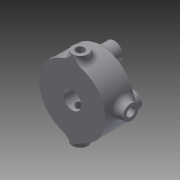
# Autodesk Inventor part: stick-holder-top
Saved by Autodesk Inventor 2014 (Build 180170000, 170)
## iProperties
Created: 2017-07-21
Part Number: stick-holder-top
Material: 一般
Document SubType Name: Modeling
Designer: hide
Density: 1 g/cm^3
Appearance: 既定
Author: hide
Autodesk Inventor part; units mm, degrees
ref_plane "YZ Plane" through (0, 0, 0) normal (1, 0, 0) x (0, 1, 0)
ref_plane "XZ Plane" through (0, 0, 0) normal (0, 1, 0) x (-1, 0, 0)
ref_plane "XY Plane" through (0, 0, 0) normal (0, 0, 1) x (1, 0, 0)
sketch "スケッチ1" plane through (0, 0, 0) normal (0, 1, 0) x (-1, 0, 0)
  circle A0 centre (0, 0) radius 15
  circle A1 centre (0, 10) radius 1.9
  circle A2 centre (-8.6603, -5) radius 1.9
  circle A3 centre (8.6603, -5) radius 1.9
  dimension "d0" = 30
  dimension "d1" = 10
  dimension "d2" = 3.8
  dimension "d5" = 360
  constraints: 4 centre point, 1 coincident, 7 other
  measures "d0" diameter of A0
  measures "d1" distance of A1.centre point (0, 0)
  measures "d2" diameter of A1
extrude "押し出し1" add sketch "スケッチ1" along normal blind 3
sketch "スケッチ2" plane through (0, 3, 0) normal (0, 1, 0) x (1, 0, 0)
  circle A0 centre (-8.6603, 5) radius 1.9 projected
  circle A1 centre (8.6603, 5) radius 1.9 projected
  circle A2 centre (0, -10) radius 1.9 projected
  circle A3 centre (-8.6603, 5) radius 3.9
  circle A4 centre (8.6603, 5) radius 3.9
  circle A5 centre (0, -10) radius 3.9
  dimension "d9" = 2
  dimension "d10" = 2
  dimension "d11" = 2
  constraints: 3 centre point, 3 coincident
  measures "d9" radial gap between concentric circles of A3 A0
  measures "d10" radial gap between concentric circles of A5 A2
  measures "d11" radial gap between concentric circles of A4 A1
extrude "押し出し2" add sketch "スケッチ2" along normal blind 6
sketch "スケッチ3" plane through (0, 0, 0) normal (0, -1, 0) x (1, 0, 0)
  circle A0 centre (0, 0) radius 15 projected
extrude "押し出し3" add sketch "スケッチ3" along normal blind 10
sketch "スケッチ4" plane through (0, 0, 0) normal (1, 0, 0) x (0, 1, 0)
  circle A0 centre (-1.5, 0) radius 3.5
  point P0 (0, 0)
  dimension "d16" = 7
  dimension "d17" = 1.5
  dimension "d18" = 0
  constraints: 1 centre point
  measures "d16" diameter of A0
  measures "d17" distance of point (0, 0) A0.centre
  measures "d18" vertical distance of A0.centre point (0, 0)
extrude "押し出し4" add sketch "スケッチ4" along normal mid plane 36
sketch "スケッチ5" plane through (18, -1.5, 0) normal (1, 0, 0) x (0, 0, -1)
  circle A0 centre (0, 0) radius 3.5 projected
  circle A1 centre (0, 0) radius 1.9
  point P0 (0, 1.5)
  dimension "d21" = 3.8
  constraints: 1 centre point, 1 coincident
  measures "d21" diameter of A1
extrude "押し出し5" cut sketch "スケッチ5" against normal blind 40 contours A1
sketch "スケッチ6" plane through (0, 0, 0) normal (0, 0, 1) x (1, 0, 0)
  circle A0 centre (0, -6.4621) radius 3.5
  point P0 (0, 0)
  dimension "d24" = 7
  constraints: 1 centre point
  measures "d24" diameter of A0
extrude "押し出し6" add sketch "スケッチ6" along normal mid plane 36
sketch "スケッチ7" plane through (0, -6.4621, 18) normal (0, 0, 1) x (1, 0, 0)
  circle A0 centre (0, 0) radius 3.5 projected
  circle A1 centre (0, 0) radius 1.9
  point P0 (0, 6.4621)
  dimension "d27" = 3.8
  constraints: 1 centre point, 1 coincident
  measures "d27" diameter of A1
extrude "押し出し7" cut sketch "スケッチ7" against normal blind 36 contours A1
fillet "フィレット1" radius 3 9 edges at (14.8649, 1.3662, 2.0087) (14.8649, 1.3662, -2.0087) (14.6723, -3.089, -3.1185) (14.6722, -3.0888, 3.1186) (-15, -5, 0.0053) (-14.8649, 1.3662, -2.0087) (-14.8649, 1.3662, 2.0087) (-3.4986, -6.3621, 14.5863) (-3.4986, -6.3621, -14.5863)
fillet "フィレット2" radius 2 3 edges at (4.7603, 3, -5) (-12.5603, 3, -5) (-3.9, 3, 10)
sketch "スケッチ8" plane through (0, 3, 0) normal (0, 1, 0) x (1, 0, 0)
  arc A0 (-14.4818, -3.9087) -> (-3.8045, -14.5095) centre (0, 0) ccw projected
  circle A1 centre (0, 0) radius 4
  dimension "d32" = 8
  constraints: 1 centre point, 1 coincident
  measures "d32" diameter of A1
extrude "押し出し8" cut sketch "スケッチ8" against normal blind 36
equation "\"d10\" = d9"
equation "\"d11\" = d9"
